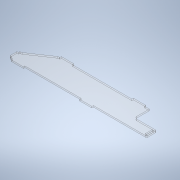
# Autodesk Inventor part: sideWallRight
Saved by Autodesk Inventor 2020 (Build 240168000, 168)
## iProperties
Created: 2020-03-02
Part Number: sideWallRight
Material: Polycarbonate, Clear
Document SubType Name: Modeling
Designer: n10208577
Density: 1.2 g/cm^3
Appearance: Polycarbonate - Clear
Author: n10208577
Autodesk Inventor part; units mm, degrees
ref_plane "YZ Plane" through (0, 0, 0) normal (1, 0, 0) x (0, 1, 0)
ref_plane "XZ Plane" through (0, 0, 0) normal (0, 1, 0) x (-1, 0, 0)
ref_plane "XY Plane" through (0, 0, 0) normal (0, 0, 1) x (1, 0, 0)
sketch "Sketch1" plane through (0, 0, 0) normal (0, 1, 0) x (-1, 0, 0)
  line L0 (4.3325, 36.172) -> (109.3325, 36.172)
  line L1 (134.3325, 36.172) -> (247.3325, 36.172)
  line L2 (277.3325, 36.172) -> (277.3325, 33.172)
  line L3 (277.3325, 33.172) -> (280.3325, 33.172)
  line L4 (280.3325, 33.172) -> (280.3325, 19.172)
  line L5 (280.3325, 19.172) -> (277.3325, 19.172)
  line L6 (277.3325, 19.172) -> (277.3325, 16.172)
  line L7 (201.8325, -13.828) -> (201.8325, -16.828)
  line L8 (201.8325, -16.828) -> (226.8325, -16.828)
  line L9 (226.8325, -16.828) -> (226.8325, -13.828)
  line L10 (56.8325, -13.828) -> (56.8325, -16.828)
  line L11 (56.8325, -16.828) -> (81.8325, -16.828)
  line L12 (81.8325, -16.828) -> (81.8325, -13.828)
  line L13 (81.8325, -13.828) -> (201.8325, -13.828)
  line L14 (56.8325, -13.828) -> (46.8325, -13.828)
  line L15 (46.8325, -13.828) -> (46.8325, 11.172)
  arc A0 (46.8325, 11.172) -> (41.8325, 16.172) centre (41.8325, 11.172) ccw
  line L16 (41.8325, 16.172) -> (4.3325, 16.172)
  arc A1 (2.3325, 18.172) -> (4.3325, 16.172) centre (4.3325, 18.172) ccw
  line L17 (2.3325, 18.172) -> (2.3325, 34.172)
  arc A2 (4.3325, 36.172) -> (2.3325, 34.172) centre (4.3325, 34.172) ccw
  line L18 (5.4325, 19.172) -> (8.2325, 19.172)
  line L19 (8.2325, 19.172) -> (8.2325, 33.172)
  line L20 (8.2325, 33.172) -> (5.4325, 33.172)
  line L21 (5.4325, 33.172) -> (5.4325, 19.172)
  line L22 (109.3325, 36.172) -> (109.3325, 39.172)
  line L23 (109.3325, 39.172) -> (134.3325, 39.172)
  line L24 (134.3325, 39.172) -> (134.3325, 36.172)
  line L25 (277.3325, 36.172) -> (272.3325, 36.172)
  line L26 (272.3325, 36.172) -> (272.3325, 39.172)
  line L27 (272.3325, 39.172) -> (247.3325, 39.172)
  line L28 (247.3325, 39.172) -> (247.3325, 36.172)
  line L29 (226.8325, -13.828) -> (228.3045, -13.828)
  line L30 (277.3325, 16.172) -> (275.8605, 16.172)
  arc A3 (275.8605, 16.172) -> (273.0655, 15.3179) centre (275.8605, 11.172) ccw
  line L31 (273.0655, 15.3179) -> (231.0995, -12.9739)
  arc A4 (228.3045, -13.828) -> (231.0995, -12.9739) centre (228.3045, -8.828) ccw
  constraints: 64 end point, 10 point on circle, 5 centre point
extrude "Extrusion1" add sketch "Sketch1" along normal blind 3
body "Solid1"
